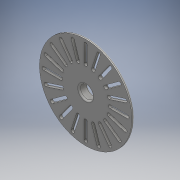
# Autodesk Inventor part: encoder wheel
Saved by Autodesk Inventor 2016 (Build 200138000, 138)
## iProperties
Created: 2016-04-18
Part Number: encoder wheel
Material: Generic
Document SubType Name: Modeling
Designer: rmainhar
Density: 1 g/cm^3
Appearance: Default
Author: rmainhar
Autodesk Inventor part; units mm, degrees
ref_plane "YZ Plane" through (0, 0, 0) normal (1, 0, 0) x (0, 1, 0)
ref_plane "XZ Plane" through (0, 0, 0) normal (0, 1, 0) x (-1, 0, 0)
ref_plane "XY Plane" through (0, 0, 0) normal (0, 0, 1) x (1, 0, 0)
sketch "Sketch1" plane through (0, 0, 0) normal (0, 1, 0) x (-1, 0, 0)
  circle A0 centre (0, 0) radius 5.5
  circle A1 centre (0, 0) radius 2.25
  circle A2 centre (0, 0) radius 16
  dimension "d0" = 11
  dimension "d1" = 4.5
  dimension "d2" = 32
  constraints: 3 centre point, 3 coincident
  measures "d0" diameter of A0
  measures "d1" diameter of A1
  measures "d2" diameter of A2
extrude "Extrusion1" add sketch "Sketch1" along normal blind 0.9 contours A2
extrude "Extrusion2" add sketch "Sketch1" along normal blind 3 contours A0
fillet "Fillet1" radius 1 1 edges at (5.5, 0.9, 0)
sketch "Sketch2" plane through (0, 0.9, 0) normal (0, 1, 0) x (1, 0, 0)
  circle A0 centre (0, 0) radius 2.25 projected
  line L0 (0, 0) -> (0, 20.2809)
  line L1 (0, 15.075) -> (0, 7.925) construction
  line L2 (0.575, 14.5) -> (0.575, 8.5)
  line L3 (-0.575, 8.5) -> (-0.575, 14.5)
  arc A1 (0.575, 14.5) -> (-0.575, 14.5) centre (0, 14.5) ccw
  arc A2 (-0.575, 8.5) -> (0.575, 8.5) centre (0, 8.5) ccw
  point P0 (0, 11.5)
  dimension "d8" = 8.5
  dimension "d9" = 14.5
  dimension "d10" = 1.15
  constraints: 10 end point, 6 point on circle, 4 point on line, 4 tangent, 2 centre point, 1 midpoint, 1 parallel, 1 vertical
  measures "d8" distance of point (0, 0) A2.centre
  measures "d9" distance of A1.centre point (0, 0)
  measures "d10" distance between parallel lines of L2 L3
extrude "Extrusion3" cut sketch "Sketch2" against normal through all contours A2 L3 A1 L0 | L0 A1 L2 A2
pattern_circular "Circular Pattern1" count 20 over 360 about axis through (0, 0, 0) along (0, 1, 0) of "Extrusion3"
fillet "Fillet2" radius 0.5 3 edges at (16, 0.9, 0) (2.25, 3, 0) (2.25, 0, 0)
body "Solid1"
